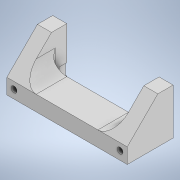
# Autodesk Inventor part: 3DPrintedPrintHeadRetainingFrame
Saved by Autodesk Inventor 2021 (Build 250183000, 183)
## iProperties
Created: 2021-10-26
Part Number: 3DPrintedPrintHeadRetainingFrame
Material: Generic
Document SubType Name: Sheet Metal
Designer: Unit-005
Density: 1 g/cm^3
Sheet Metal Rule: Default
Appearance: Default
Author: Unit-005
## iProperties of the stored document _3DPrint.ipt
Created: 2021-10-26
Part Number: _3DPrint
Material: Generic
Document SubType Name: Modeling
Designer: Unit-005
Density: 1 g/cm^3
Appearance: Default
Author: Unit-005
Autodesk Inventor part; units mm, degrees
ref_plane "YZ Plane" through (0, 0, 0) normal (1, 0, 0) x (0, 1, 0)
ref_plane "XZ Plane" through (0, 0, 0) normal (0, 1, 0) x (-1, 0, 0)
ref_plane "XY Plane" through (0, 0, 0) normal (0, 0, 1) x (1, 0, 0)
sketch "Sketch1" plane through (0, 0, 0) normal (0, 0, 1) x (1, 0, 0)
  line L0 (-50.0126, 6.35) -> (50.0126, 6.35)
  line L1 (50.0126, 6.35) -> (50.0126, -6.35)
  line L2 (50.0126, -6.35) -> (-50.0126, -6.35)
  line L3 (-50.0126, -6.35) -> (-50.0126, 6.35)
  line L4 (-50.0126, 6.35) -> (50.0126, -6.35) construction
  line L5 (50.0126, 6.35) -> (-50.0126, -6.35) construction
  point P0 (0, 0)
  dimension "d0" = 100.0252
  dimension "d1" = 12.7
  constraints: 12 end point, 2 midpoint, 2 parallel, 1 horizontal, 1 perpendicular
  measures "d0" distance of L1.end L2.end
  measures "d1" distance of L0.end L1.end
extrude "Extrusion1" add sketch "Sketch1" along normal blind 25.4
sketch "Sketch2" plane through (0, 0, 0) normal (0, 0, 1) x (1, 0, 0)
  line L0 (-50.0126, -6.35) -> (50.0126, -6.35) projected
  line L1 (-50.0126, 6.35) -> (-50.0126, -6.35) projected
  line L2 (50.0126, 6.35) -> (-50.0126, 6.35) projected
  line L3 (50.0126, -6.35) -> (50.0126, 6.35) projected
  line L4 (-70.0176, 0) -> (70.0176, 0) projected
  line L5 (0, -8.89) -> (0, 8.89) projected
  line L6 (50.0126, -6.35) -> (50.0126, 6.35) projected
  line L7 (-50.0126, -6.35) -> (50.0126, -6.35) projected
  line L8 (50.0126, 6.35) -> (38.3286, 6.35)
  line L9 (38.3286, 6.35) -> (38.3286, -6.35)
  line L10 (38.3286, -6.35) -> (50.0126, -6.35)
  line L11 (50.0126, -6.35) -> (50.0126, 6.35)
  point P0 (0, 0)
  point P1 (38.3286, 6.35)
  point P2 (38.3286, -6.35)
  dimension "d4" = 11.684
  constraints: 8 end point, 2 parallel, 1 horizontal, 1 perpendicular, 1 point on line
  measures "d4" distance of L10.end L9.end
extrude "Extrusion2" add sketch "Sketch2" against normal blind 12.7 contours L9 L4 L3 L0 | L9 L2 L3 L4
mirror "Mirror1" about plane through (0, 0, 0) normal (1, 0, 0) of "Extrusion2"
fillet "Fillet1" radius 3.175 2 edges at (38.3286, 0, 0) (-38.3286, 0, 0)
sketch "Sketch3" plane through (0, 0, 0) normal (0, 0, -1) x (-1, 0, 0)
  line L0 (70.0176, 0) -> (-70.0176, 0) projected
  line L1 (0, -8.89) -> (0, 8.89) projected
  line L2 (35.1536, 6.35) -> (35.1536, -6.35) projected
  line L3 (-35.1536, 6.35) -> (35.1536, 6.35) projected
  line L4 (-35.1536, -6.35) -> (-35.1536, 6.35) projected
  line L5 (35.1536, -6.35) -> (-35.1536, -6.35) projected
  circle A0 centre (0, -4.1402) radius 2.0574
  point P0 (0, 0)
  dimension "d9" = 4.1148
  dimension "d10" = 2.2098
  constraints: 1 centre point, 1 point on line
  measures "d9" diameter of A0
  measures "d10" distance from line of L5 A0.centre
extrude "Extrusion3" cut sketch "Sketch3" against normal blind 1.5875 contours A0 L1 | L1 A0
pattern_linear "Rectangular Pattern1" count 11 spacing 6.35 along (1, 0, 0) of "Extrusion3" first direction both ways yes
sketch "Sketch4" plane through (0, 0, -12.7) normal (0, 0, -1) x (-1, 0, 0)
  line L0 (70.0176, 0) -> (-70.0176, 0) projected
  line L1 (0, -8.89) -> (0, 8.89) projected
  line L2 (-50.0126, -6.35) -> (-38.3286, -6.35) projected
  line L3 (-38.3286, -6.35) -> (-38.3286, 6.35) projected
  line L4 (-38.3286, 6.35) -> (-50.0126, 6.35) projected
  line L5 (-50.0126, 6.35) -> (-50.0126, -6.35) projected
  line L6 (50.0126, -6.35) -> (38.3286, -6.35) projected
  line L7 (50.0126, 6.35) -> (50.0126, -6.35) projected
  line L8 (38.3286, 6.35) -> (50.0126, 6.35) projected
  line L9 (38.3286, -6.35) -> (38.3286, 6.35) projected
  line L10 (-38.3286, -6.35) -> (-38.3286, 6.35) projected
  line L11 (-38.3286, 3.683) -> (-39.3446, 3.683)
  line L12 (-39.3446, 3.683) -> (-39.3446, -5.842)
  line L13 (-39.3446, -5.842) -> (-38.3286, -5.842)
  line L14 (-38.3286, -5.842) -> (-38.3286, 3.683)
  point P0 (0, 0)
  point P1 (-38.3286, 3.683)
  dimension "d19" = 1.016
  dimension "d20" = 9.525
  dimension "d21" = 0.508
  constraints: 8 end point, 2 parallel, 1 horizontal, 1 perpendicular, 1 point on line
  measures "d19" distance of L13.end L12.end
  measures "d20" distance of L12.end L11.end
  measures "d21" distance between parallel lines of L2 L13
extrude "Extrusion4" cut sketch "Sketch4" against normal blind 6.35 contours L3 L13 L12 L0 | L0 L12 L11 L3
mirror "Mirror2" about plane through (0, 0, 0) normal (1, 0, 0) of "Extrusion4"
sketch "Sketch5" plane through (0, 0, -12.7) normal (0, 0, -1) x (-1, 0, 0)
  line L0 (-38.3286, -5.842) -> (-39.3446, -5.842) projected
  line L1 (-39.3446, -5.842) -> (-39.3446, 3.683) projected
  line L2 (-39.3446, 3.683) -> (-38.3286, 3.683) projected
  line L3 (-38.3286, 3.683) -> (-38.3286, 6.35) projected
  line L4 (-38.3286, 6.35) -> (-50.0126, 6.35) projected
  line L5 (-50.0126, 6.35) -> (-50.0126, -6.35) projected
  line L6 (-50.0126, -6.35) -> (-38.3286, -6.35) projected
  line L7 (-38.3286, -6.35) -> (-38.3286, -5.842) projected
  line L8 (47.9806, -6.35) -> (47.9806, 6.35) projected
  line L9 (50.0126, 6.35) -> (50.0126, -6.35) projected
  line L10 (38.3286, 3.683) -> (39.3446, 3.683) projected
  line L11 (39.3446, 3.683) -> (39.3446, -5.842) projected
  line L12 (39.3446, -5.842) -> (38.3286, -5.842) projected
  line L13 (38.3286, -6.35) -> (38.3286, -5.842) projected
  line L14 (50.0126, -6.35) -> (38.3286, -6.35) projected
  line L15 (50.0126, 6.35) -> (50.0126, -6.35) projected
  line L16 (38.3286, 6.35) -> (50.0126, 6.35) projected
  line L17 (38.3286, 3.683) -> (38.3286, 6.35) projected
  line L18 (70.0176, 0) -> (-70.0176, 0) projected
  line L19 (0, -8.89) -> (0, 8.89) projected
  circle A0 centre (-44.0182, 0.6604) radius 3.3782
  point P0 (0, 0)
  dimension "d24" = 6.7564
  dimension "d25" = 7.0104
  dimension "d26" = 5.9944
  constraints: 1 centre point
  measures "d24" diameter of A0
  measures "d25" distance from line of L6 A0.centre
  measures "d26" distance from line of L5 A0.centre
hole "Hole1" at (44.0182, 0.6604, -12.7) direction (0, 0, 1) diameter 4.9276 end through all clearance for "Socket Head Cap Screw" size "#8" standard "Ansi Unified Screw Threads"
mirror "Mirror3" about plane through (0, 0, 0) normal (1, 0, 0) of "Hole1"
sketch "Sketch6" plane through (38.3286, 6.35, -12.7) normal (0, 1, 0) x (1, 0, 0)
  line L0 (11.684, -38.1) -> (-88.3412, -38.1) projected
  line L1 (11.684, 0) -> (11.684, -38.1) projected
  line L2 (0, 0) -> (11.684, 0) projected
  line L3 (0, -9.525) -> (0, 0) projected
  arc A0 (-3.175, -12.7) -> (0, -9.525) centre (-3.175, -9.525) ccw projected
  line L4 (-3.175, -12.7) -> (-73.4822, -12.7) projected
  arc A1 (-76.6572, -9.525) -> (-73.4822, -12.7) centre (-73.4822, -9.525) ccw projected
  line L5 (-76.6572, -9.525) -> (-76.6572, 0) projected
  line L6 (-76.6572, 0) -> (-88.3412, 0) projected
  line L7 (-88.3412, 0) -> (-88.3412, -38.1) projected
  line L8 (-108.397, -12.7) -> (31.9938, -12.7) projected
  line L9 (-38.3286, 7.62) -> (-38.3286, -45.72) projected
  line L10 (0, -9.525) -> (0, 0) projected
  line L11 (0, 0) -> (11.684, 0)
  line L12 (11.684, 0) -> (11.684, -38.1)
  line L13 (11.684, -38.1) -> (0, -38.1)
  line L14 (0, -38.1) -> (0, 0)
  line L15 (-88.3412, 0) -> (-88.3412, -38.1)
  line L16 (-76.6572, 0) -> (-88.3412, 0)
  line L17 (-76.6572, -9.525) -> (-76.6572, 0)
  arc A2 (-76.6572, -9.525) -> (-73.4822, -12.7) centre (-73.4822, -9.525) ccw
  line L18 (-76.6572, -9.525) -> (-76.6572, 0)
  line L19 (-76.6572, 0) -> (-88.3412, 0)
  line L20 (-88.3412, 0) -> (-88.3412, -38.1)
  line L21 (-88.3412, -38.1) -> (-76.6572, -38.1)
  line L22 (-76.6572, -38.1) -> (-76.6572, 0)
  point P0 (-38.3286, -12.7)
  constraints: 24 end point, 5 symmetric about line, 2 collinear, 2 parallel, 2 point on circle, 1 centre point, 1 horizontal, 1 perpendicular, 1 other
extrude "Extrusion5" add sketch "Sketch6" along normal blind 25.4 contours L0 L14 L8 L1 | L8 L14 L3 L2 L1 | L0 L7 L8 L22 | L8 L7 L6 L5 L22
chamfer "Chamfer2" distance 25.4 angle 45 2 edges at (44.1706, 31.75, 25.4) (-44.1706, 31.75, 25.4)
fillet "Fillet3" radius 12.7 2 edges at (38.3286, 6.35, 11.1125) (-38.3286, 6.35, 11.1125)
equation "\"d32\" = Thickness"
equation "\"BendRadius\" = Thickness"
equation "\"BendReliefWidth\" = Thickness"
equation "\"BendReliefDepth\" = 0.5 * Thickness"
equation "\"CornerReliefSize\" = 4 * Thickness"
equation "\"MinimumRemnant\" = 2 * Thickness"
equation "\"TransitionRadius\" = BendRadius"
equation "\"JacobiRadiusSize\" = BendRadius"
equation "\"GapSize\" = Thickness"
equation "\"Thickness\" = 3.048"
body "Solid1"
